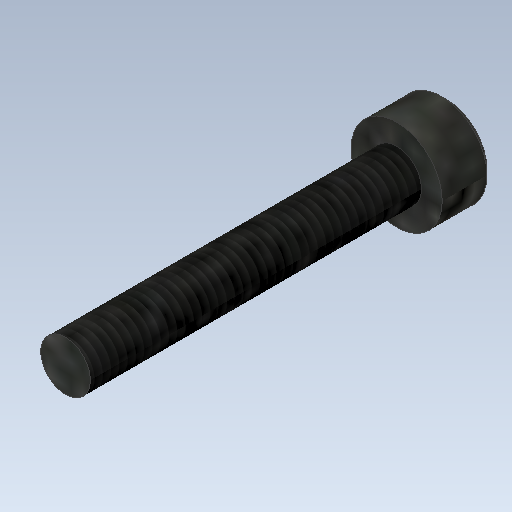
# Autodesk Inventor part: キャップボルトM3×20
Saved by Autodesk Inventor 2020 (Build 240168000, 168)
## iProperties
Created: 2019-05-02
Part Number: キャップボルトM3×20
Material: 鋼
Document SubType Name: Modeling
Designer: tanjihayato
Density: 7.85 g/cm^3
Appearance: プレート
Mass: 1.60816 g
Surface Area: 2.95953 cm^2
Volume: 0.204861 cm^3
Author: tanjihayato
Autodesk Inventor part; units mm, degrees
ref_plane "YZ Plane" through (0, 0, 0) normal (1, 0, 0) x (0, 1, 0)
ref_plane "XZ Plane" through (0, 0, 0) normal (0, 1, 0) x (-1, 0, 0)
ref_plane "XY Plane" through (0, 0, 0) normal (0, 0, 1) x (1, 0, 0)
sketch "スケッチ1" plane through (0, 0, 0) normal (0, 0, 1) x (1, 0, 0)
  circle A0 centre (0, 0) radius 2.75
  circle A1 centre (0, 0) radius 1.5
  dimension "d0" = 5.5
  dimension "d1" = 3
  constraints: 2 centre point, 2 coincident
  measures "d0" diameter of A0
  measures "d1" diameter of A1
extrude "押し出し1" add sketch "スケッチ1" along normal blind 3
extrude "押し出し2" add sketch "スケッチ1" along normal blind 23 contours A1
chamfer "面取り1" distance 0.3 angle 45 1 edges at (-2.75, 0, 0)
sketch "スケッチ2" plane through (0, 0, 0) normal (0, 0, -1) x (-1, 0, 0)
  line L0 (0, -1.4434) -> (-1.25, -0.7217)
  line L1 (-1.25, -0.7217) -> (-1.25, 0.7217)
  line L2 (-1.25, 0.7217) -> (0, 1.4434)
  line L3 (0, 1.4434) -> (1.25, 0.7217)
  line L4 (1.25, 0.7217) -> (1.25, -0.7217)
  line L5 (1.25, -0.7217) -> (0, -1.4434)
  point P0 (0, 0)
  point P1 (0, 0)
  dimension "d9" = 2.5
  constraints: 12 end point, 1 coincident, 1 vertical, 13 other
  measures "d9" distance between parallel lines of L2 L5
extrude "押し出し3" cut sketch "スケッチ2" against normal blind 1.3
thread "ねじ1" size "M3x0.5" class "6g" standard "ANSI Metric M Profile" full length
